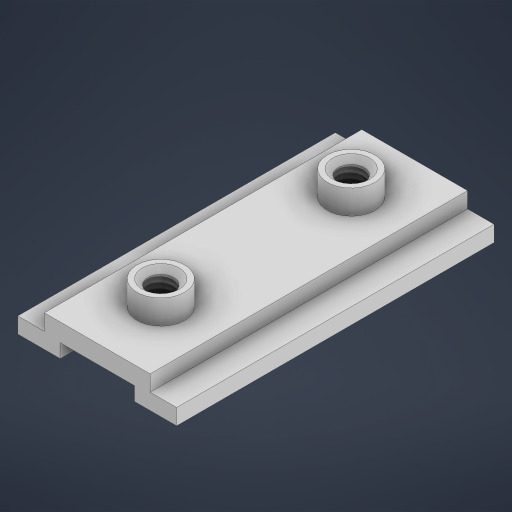
# Autodesk Inventor part: Igus Gleiter
Saved by Autodesk Inventor 2024.2 (Build 282272000, 272)
## iProperties
Created: 2023-12-02
Part Number: Igus Gleiter
Material: Generisch
Document SubType Name: Modeling
Designer: jacob
Density: 1 g/cm^3
Appearance: Vorgabe
Author: jacob
Autodesk Inventor part; units mm, degrees
ref_plane "YZ Plane" through (0, 0, 0) normal (1, 0, 0) x (0, 1, 0)
ref_plane "XZ Plane" through (0, 0, 0) normal (0, 1, 0) x (-1, 0, 0)
ref_plane "XY Plane" through (0, 0, 0) normal (0, 0, 1) x (1, 0, 0)
sketch "Skizze1" plane through (0, 0, 0) normal (0, 0, 1) x (1, 0, 0)
  line L0 (0, 0) -> (0, 1.7)
  line L1 (0, 1.7) -> (-5, 1.7)
  line L2 (-5, 1.7) -> (-5, 0.2)
  line L3 (-5, 0.2) -> (-7.5, 0.2)
  line L4 (-7.5, 0.2) -> (-7.5, -1.3)
  line L5 (-7.5, -1.3) -> (-3.5, -1.3)
  line L6 (-3.5, -1.3) -> (-3.5, 0)
  line L7 (-3.5, 0) -> (0, 0)
  dimension "d0" = 4
  dimension "d1" = 1.5
  dimension "d2" = 2.5
  dimension "d3" = 3
  dimension "d4" = 5
  dimension "d5" = 1.7
  constraints: 16 end point, 7 perpendicular, 1 vertical
  measures "d0" distance of L4.end L5.end
  measures "d1" distance of L3.end L4.end
  measures "d2" distance of L2.end L3.end
  measures "d3" distance between parallel lines of L5 L1
  measures "d4" distance of L0.end L1.end
  measures "d5" distance of L0.start L0.end
extrude "Extrusion1" add sketch "Skizze1" along normal blind 30
mirror "Spiegeln1" about plane through (0, 0, 0) normal (1, 0, 0) of "Extrusion1"
sketch "Skizze2" plane through (-5, 1.7, 30) normal (0, 1, 0) x (1, 0, 0)
  circle A0 centre (5, 24) radius 2.25
  circle A1 centre (5, 6) radius 2.25
  line L0 (10, 30) -> (0, 30) projected
  line L1 (5, 30) -> (5, 24) construction
  line L2 (5, 6) -> (5, 0) construction
  line L3 (0, 0) -> (10, 0) construction
  dimension "d8" = 4.5
  dimension "d9" = 18
  constraints: 4 end point, 2 centre point, 2 midpoint, 2 vertical alignment, 1 collinear, 1 equal radius, 1 vertical
  measures "d8" diameter of A1
  measures "d9" distance of L2.start L1.end
extrude "Extrusion2" add sketch "Skizze2" along normal blind 2.3
sketch "Skizze3" plane through (0, 4, 24) normal (0, 1, 0) x (1, 0, 0)
  circle A0 centre (0, 0) radius 2.25 construction
  circle A1 centre (0, 18) radius 2.25 construction
  point P0 (0, 24)
  constraints: 2 coincident
hole "Bohrung1" at (0, 4, 24) at (0, 4, 6) direction (0, -1, 0) diameter 2.459 end through all countersink diameter 3.5 countersink angle 90 thread size "M3x0.5" class "6H" standard "ISO Metric profile"
